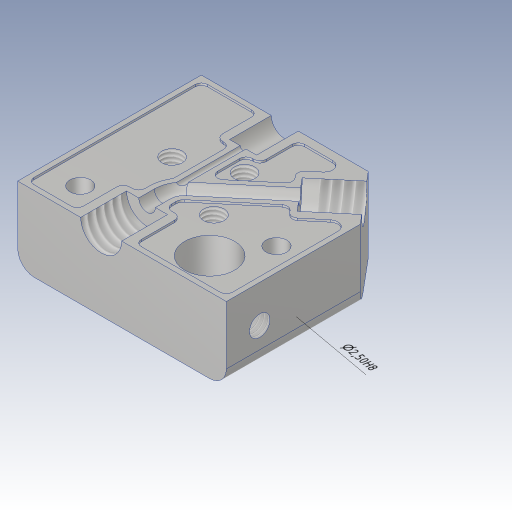
# Autodesk Inventor part: BT001_huenin20_23
Saved by Autodesk Inventor 2023.3 (Build 273359000, 359)
## iProperties
Company: HTBLA Kaindorf
RuleStatus: InUse
Created: 2023-05-23
Part Number: BT001_huenin20_23
Project: Fiberprinter-Hotend
Material: Aluminium
Description: Heizblock_Seite1
Document SubType Name: Modeling
Designer: huenin20
Density: 2.7 g/cm^3
Appearance: Aluminium - flach
Mass: 10.9063 g
Surface Area: 24.2904 cm^2
Volume: 4.03936 cm^3
AfterDocNew0: iProperties-Editor_aufrufen
Author: nicob
Keywords: 2023
Autodesk Inventor part; units mm, degrees
ref_plane "YZ Plane" through (0, 0, 0) normal (1, 0, 0) x (0, 1, 0)
ref_plane "XZ Plane" through (0, 0, 0) normal (0, 1, 0) x (-1, 0, 0)
ref_plane "XY Plane" through (0, 0, 0) normal (0, 0, 1) x (1, 0, 0)
sketch "Skizze3" plane through (0, 0, 0) normal (0, 0, 1) x (1, 0, 0)
  line L0 (0, 0) -> (-22, 0)
  line L1 (-16.0412, 25) -> (0, 25)
  line L2 (0, 25) -> (0, 0)
  circle A0 centre (-4, 19) radius 3
  line L3 (-22, 20) -> (-16.0412, 25)
  line L4 (-22, 20) -> (-22, 0)
  line L5 (-19.0206, 22.5) -> (-9.2812, 10.893)
  arc A1 (-9.2812, 10.893) -> (-7.3661, 10) centre (-7.3661, 12.5) ccw
  line L6 (-7.3661, 10) -> (0, 10)
  dimension "d115" = 6
  dimension "d116" = 6
  dimension "d117" = 4
  dimension "d234" = 130
  dimension "d236" = 25
  dimension "d237" = 22
  dimension "d238" = 2.5
  dimension "d306" = 15
  dimension "d325" = 20
  constraints: 15 end point, 2 centre point, 2 perpendicular, 2 point on circle, 2 tangent, 1 horizontal, 1 midpoint, 1 parallel, 1 point on line
  measures "d115" diameter of A0
  measures "d116" distance from line of L1 A0.centre
  measures "d117" distance from line of L2 A0.centre
  measures "d234" angle of L4 L3
  measures "d236" distance between parallel lines of L1 L0
  measures "d237" distance between parallel lines of L2 L4
  measures "d238" radius of A1
  measures "d306" distance between parallel lines of L1 L6
  measures "d325" distance of L3.start L0.end
extrude "Extrusion11" add sketch "Skizze3" against normal blind 9
sketch "Skizze19" plane through (-22, 20, -9) normal (-0.6427876, 0.7660444, 0) x (0.7660444, 0.6427876, 0)
  circle A0 centre (3.8893, -9) radius 1
  point P0 (3.9972, -9)
  dimension "d241" = 2
  constraints: 1 centre point, 1 coincident
  measures "d241" diameter of A0
sweep "Sweeping4" cut profiles "Skizze19" path "Skizze3" path curves L5 A1 L6
hole "Bohrung17" at (-19.0206, 22.5, 0) direction (0.6427876, -0.7660444, 0) diameter 4.917 depth 5.5
sketch "Skizze20" plane through (0, 0, -9) normal (1, 0, 0) x (0, 0, -1)
  arc A0 (-9, 9) -> (-9, 11) centre (-9, 10) ccw projected
  point P0 (-9, 0)
hole "Bohrung18" at (0, 10, 0) direction (-1, 0, 0) diameter 4.917 depth 5.5
hole "Bohrung27" at (0, 10, 0) direction (-1, 0, 0) diameter 0.7 depth 11
sketch "Skizze21" plane through (-22, 0, 0) normal (-1, 0, 0) x (0, 0, 1)
  arc A0 (0, 11) -> (0, 9) centre (0, 10) ccw projected
  line L0 (0, 20) -> (0, 0) projected
  line L1 (0, 10.35) -> (-0.35, 10)
  line L2 (-0.35, 10) -> (0, 9.65)
  line L3 (0, 9.65) -> (0, 10.35) projected
  arc A1 (0, 10.35) -> (0, 9.65) centre (0, 10) ccw projected
  point P0 (0, 10)
  point P1 (-0.35, 10)
  point P2 (-0.35, 10)
  point P3 (0, 9.65)
  dimension "d345" = 45
  dimension "d347" = 0.7
  constraints: 4 end point, 2 point on line, 1 horizontal alignment, 1 midpoint, 1 perpendicular
  measures "d345" angle of L0 L2
  measures "d347" distance of L1.start L2.end
hole "Bohrung20" at (-22, 10, 0) direction (1, 0, 0) diameter 3.242 depth 5
sketch "Skizze22" plane through (0, 0, 0) normal (0, 0, 1) x (1, 0, 0)
  line L0 (0, 7.5415) -> (-5.5, 7.5415) projected
  line L1 (0, 12.4585) -> (0, 7.5415) projected
  line L2 (-5.5, 12.4585) -> (0, 12.4585) projected
  line L3 (-5.5, 7.5415) -> (-5.5, 12.4585) projected
  line L4 (-5.5, 10) -> (-7.3661, 10)
  line L5 (-7.3661, 9) -> (-7.3661, 11) projected
  line L6 (-6, 10) -> (-6, 11.5)
  line L7 (-6, 11.5) -> (-7, 11.5)
  line L8 (-7, 11.5) -> (-7, 10)
  point P0 (0, 0)
  dimension "d273" = 1
  dimension "d274" = 0.5
  dimension "d275" = 3
  constraints: 8 end point, 2 midpoint, 2 perpendicular, 2 point on line, 1 vertical
  measures "d273" distance of L6.end L7.end
  measures "d274" distance between parallel lines of L3 L6
  measures "d275" diameter of L7 L4
revolve "Umdrehung2" [suppressed]
sketch "Skizze23" plane through (0, 25, -9) normal (0, 1, 0) x (0, 0, -1)
  line L0 (0, 7) -> (0, 1) projected
  line L1 (-9, 1) -> (-9, 7) projected
  line L2 (-9, 0) -> (0, 0) projected
  point P0 (-4.5, 4)
  point P1 (-9, 4)
  point P2 (-4.5, 0)
  constraints: 2 midpoint, 1 horizontal alignment, 1 vertical alignment
hole "Bohrung28" at (-4, 25, -4.5) direction (0, -1, 0) diameter 2.459 depth 6 tip angle 118
sketch "Skizze24" plane through (0, 0, 0) normal (0, 0, 1) x (1, 0, 0)
  line L0 (-7.3661, 11) -> (-5.5, 11) projected
  line L1 (-5.5, 11) -> (-5.5, 12.4585) projected
  line L2 (-5.5, 12.4585) -> (0, 12.4585) projected
  line L3 (0, 12.4585) -> (0, 25) projected
  line L4 (0, 25) -> (-16.0412, 25) projected
  circle A0 centre (-4, 19) radius 3 projected
  line L5 (-16.0412, 25) -> (-17.1373, 24.0803) projected
  line L6 (-17.1373, 24.0803) -> (-13.602, 19.867) projected
  line L7 (-13.602, 19.867) -> (-14.7192, 18.9295) projected
  line L8 (-14.7192, 18.9295) -> (-8.5152, 11.5358) projected
  arc A1 (-8.5152, 11.5358) -> (-7.3661, 11) centre (-7.3661, 12.5) ccw projected
  line L9 (-5.5, 9) -> (-7.3661, 9) projected
  arc A2 (-9.3977, 9.65) -> (-7.3661, 9) centre (-7.3661, 12.5) ccw projected
  line L10 (-10.131, 10.35) -> (-16.2513, 17.644) projected
  line L11 (-16.2513, 17.644) -> (-17.3686, 16.7065) projected
  line L12 (-17.3686, 16.7065) -> (-20.9039, 20.9197) projected
  line L13 (-20.9039, 20.9197) -> (-22, 20) projected
  line L14 (-22, 20) -> (-22, 11.621) projected
  line L15 (-22, 11.621) -> (-17, 11.621) projected
  line L16 (-17, 11.621) -> (-17, 8.379) projected
  line L17 (-17, 8.379) -> (-22, 8.379) projected
  line L18 (-22, 8.379) -> (-22, 0) projected
  line L19 (-22, 0) -> (0, 0) projected
  line L20 (0, 0) -> (0, 7.5415) projected
  line L21 (0, 7.5415) -> (-5.5, 7.5415) projected
  line L22 (-5.5, 7.5415) -> (-5.5, 9) projected
  line L23 (-9.3977, 9.65) -> (-11, 9.65) projected
  line L24 (-11, 9.65) -> (-11, 10.35) projected
  line L25 (-11, 10.35) -> (-10.131, 10.35) projected
  point P0 (-14.7, 12.48)
  point P1 (-9, 22)
  point P2 (-8.5, 15)
  point P3 (-12, 6.5)
  point P4 (-3.5, 4)
  dimension "d343" = 7.3
  dimension "d344" = 13
  dimension "d357" = 6.5
  dimension "d358" = 10
  dimension "d359" = 4
  dimension "d360" = 3.5
  dimension "d381" = 12.48
  dimension "d382" = 3
  dimension "d383" = 10
  dimension "d384" = 8.5
  measures "d343" distance from line of L14 point (-14.7, 12.48)
  measures "d344" distance from line of L14 point (-9, 22)
  measures "d357" distance from line of L19 point (-12, 6.5)
  measures "d358" distance from line of L18 point (-12, 6.5)
  measures "d359" distance from line of L19 point (-3.5, 4)
  measures "d360" distance from line of L20 point (-3.5, 4)
  measures "d381" distance from line of L19 point (-14.7, 12.48)
  measures "d382" distance from line of L4 point (-9, 22)
  measures "d383" distance from line of L4 point (-8.5, 15)
  measures "d384" distance from line of L3 point (-8.5, 15)
hole "Bohrung23" at (-9, 22, 0) at (-3.5, 4, 0) direction (0, 0, -1) diameter 2.5 end through all
fillet "Rundung5" radius 2 2 edges at (-11, 0, -9) (-8.0206, 25, -9)
hole "Bohrung24" at (-8.5, 15, 0) at (-12, 6.5, 0) at (-14.7, 12.48, 0) direction (0, 0, -1) diameter 2.459 end through all
sketch "Skizze25" plane through (-22, 20, -9) normal (-1, 0, 0) x (0, 0, 1)
  arc A0 (0, -18) -> (2, -20) centre (2, -18) ccw projected
  line L0 (9, -20) -> (2, -20) projected
  line L1 (9, -11.621) -> (9, -20) projected
  arc A1 (9, -8.379) -> (9, -11.621) centre (9, -10) ccw projected
  line L2 (9, 0) -> (9, -8.379) projected
  line L3 (9, 0) -> (0, 0) projected
  line L4 (0, -18) -> (0, 0) projected
  line L5 (2.5, -16) -> (2.5, -4) construction
  point P0 (9, -20)
  point P1 (2.5, -10)
  point P2 (2.5, -10)
  dimension "d326" = 4
  dimension "d327" = 4
  dimension "d328" = 2.5
  dimension "d361" = 0
  constraints: 2 coincident, 2 end point, 1 midpoint, 1 vertical, 1 vertical alignment
  measures "d326" distance from line of L0 L5.start
  measures "d327" distance from line of L3 point (2.5, -4)
  measures "d328" distance from line of L4 point (2.5, -4)
  measures "d361" distance from line of L5 point (2.5, -10)
hole "Bohrung25" at (-22, 4, -6.5) at (-22, 16, -6.5) direction (1, 0, 0) diameter 2.5 depth 3.5
hole "Bohrung26" at (-22, 10, -6.5) direction (1, 0, 0) diameter 1.567 depth 4 tip angle 118
extrude "Extrusion12" cut sketch "Skizze21" against normal blind 15 contours L0 L2 L1 | L1 A1 | A1 L2
sketch "Skizze27" plane through (0, 0, 0) normal (0, 0, 1) x (1, 0, 0)
  line L0 (-5.5, 11) -> (-5.5, 12.4585) projected
  line L1 (-5.5, 12.4585) -> (0, 12.4585) projected
  line L2 (0, 12.4585) -> (0, 25) projected
  line L3 (0, 25) -> (-16.0412, 25) projected
  line L4 (-16.0412, 25) -> (-17.1373, 24.0803) projected
  line L5 (-17.1373, 24.0803) -> (-13.602, 19.867) projected
  line L6 (-13.602, 19.867) -> (-14.7192, 18.9295) projected
  line L7 (-14.7192, 18.9295) -> (-8.5152, 11.5358) projected
  arc A0 (-8.5152, 11.5358) -> (-7.3661, 11) centre (-7.3661, 12.5) ccw projected
  line L8 (-7.3661, 11) -> (-5.5, 11) projected
  line L9 (-9.3977, 9.65) -> (-17, 9.65) projected
  line L10 (-17, 9.65) -> (-17, 8.379) projected
  line L11 (-17, 8.379) -> (-22, 8.379) projected
  line L12 (-22, 8.379) -> (-22, 0) projected
  line L13 (-22, 0) -> (0, 0) projected
  line L14 (0, 0) -> (0, 7.5415) projected
  line L15 (0, 7.5415) -> (-5.5, 7.5415) projected
  line L16 (-5.5, 7.5415) -> (-5.5, 9) projected
  line L17 (-5.5, 9) -> (-7.3661, 9) projected
  arc A1 (-9.3977, 9.65) -> (-7.3661, 9) centre (-7.3661, 12.5) ccw projected
  line L18 (-17, 10.35) -> (-10.131, 10.35) projected
  line L19 (-10.131, 10.35) -> (-16.2513, 17.644) projected
  line L20 (-16.2513, 17.644) -> (-17.3686, 16.7065) projected
  line L21 (-17.3686, 16.7065) -> (-20.9039, 20.9197) projected
  line L22 (-20.9039, 20.9197) -> (-22, 20) projected
  line L23 (-22, 20) -> (-22, 11.621) projected
  line L24 (-22, 11.621) -> (-17, 11.621) projected
  line L25 (-17, 11.621) -> (-17, 10.35) projected
  circle A2 centre (-14.7, 12.48) radius 1.2295 projected
  line L26 (-20.65, 7.379) -> (-17.15, 7.379)
  line L27 (-16.4, 8.129) -> (-16.4, 8.3)
  line L28 (-15.65, 9.05) -> (-9.7915, 9.05)
  arc A3 (-9.4164, 8.9495) -> (-7.3661, 8.4) centre (-7.3661, 12.5) ccw
  line L29 (-7.3661, 8.4) -> (-6.85, 8.4)
  line L30 (-6.1, 7.65) -> (-6.1, 7.2915)
  line L31 (-5.35, 6.5415) -> (-1.35, 6.5415)
  line L32 (-0.6, 5.7915) -> (-0.6, 1.35)
  line L33 (-1.35, 0.6) -> (-20.65, 0.6)
  line L34 (-21.4, 1.35) -> (-21.4, 6.629)
  line L35 (-21, 13.371) -> (-21, 19.5337)
  line L36 (-21, 19.5337) -> (-21.0272, 19.5109)
  line L37 (-21.0272, 19.5109) -> (-18.2311, 16.1786)
  line L38 (-17.1744, 16.0861) -> (-16.8998, 16.3166)
  line L39 (-15.8432, 16.2241) -> (-12.4515, 12.1821)
  line L40 (-13.026, 10.95) -> (-15.65, 10.95)
  line L41 (-16.4, 11.7) -> (-16.4, 11.871)
  line L42 (-17.15, 12.621) -> (-20.25, 12.621)
  line L43 (-8.0555, 11.9215) -> (-13.3918, 18.2811)
  line L44 (-13.2994, 19.3377) -> (-13.0248, 19.5681)
  line L45 (-12.9323, 20.6247) -> (-15.9856, 24.2635)
  line L46 (-15.9856, 24.2635) -> (-15.8228, 24.4)
  line L47 (-15.8228, 24.4) -> (-1.35, 24.4)
  line L48 (-0.6, 23.65) -> (-0.6, 14.2085)
  line L49 (-1.35, 13.4585) -> (-5.35, 13.4585)
  line L50 (-6.1, 12.7085) -> (-6.1, 12.35)
  line L51 (-6.85, 11.6) -> (-7.3661, 11.6)
  arc A4 (-8.0555, 11.9215) -> (-7.3661, 11.6) centre (-7.3661, 12.5) ccw
  arc A5 (-19.234, 17.3738) -> (-21, 16.731) centre (-20, 16.731) ccw
  arc A6 (-13.9556, 24.4) -> (-14.7217, 22.7572) centre (-13.9556, 23.4) ccw
  arc A7 (-16.4, 11.7) -> (-15.65, 10.95) centre (-15.65, 11.7) ccw
  arc A8 (-13.026, 10.95) -> (-12.4515, 12.1821) centre (-13.026, 11.7) ccw
  arc A9 (-15.8432, 16.2241) -> (-16.8998, 16.3166) centre (-16.4177, 15.742) ccw
  arc A10 (-21, 13.371) -> (-20.25, 12.621) centre (-20.25, 13.371) ccw
  arc A11 (-13.2994, 19.3377) -> (-13.3918, 18.2811) centre (-12.8173, 18.7631) ccw
  arc A12 (-6.85, 11.6) -> (-6.1, 12.35) centre (-6.85, 12.35) ccw
  arc A13 (-1.35, 13.4585) -> (-0.6, 14.2085) centre (-1.35, 14.2085) ccw
  arc A14 (-0.6, 23.65) -> (-1.35, 24.4) centre (-1.35, 23.65) ccw
  arc A15 (-6.1, 7.65) -> (-6.85, 8.4) centre (-6.85, 7.65) ccw
  arc A16 (-9.4164, 8.9495) -> (-9.7915, 9.05) centre (-9.7915, 8.3) ccw
  arc A17 (-15.65, 9.05) -> (-16.4, 8.3) centre (-15.65, 8.3) ccw
  arc A18 (-20.65, 7.379) -> (-21.4, 6.629) centre (-20.65, 6.629) ccw
  arc A19 (-21.4, 1.35) -> (-20.65, 0.6) centre (-20.65, 1.35) ccw
  arc A20 (-1.35, 0.6) -> (-0.6, 1.35) centre (-1.35, 1.35) ccw
  arc A21 (-0.6, 5.7915) -> (-1.35, 6.5415) centre (-1.35, 5.7915) ccw
  arc A22 (-6.1, 7.2915) -> (-5.35, 6.5415) centre (-5.35, 7.2915) ccw
  arc A23 (-17.15, 7.379) -> (-16.4, 8.129) centre (-17.15, 8.129) ccw
  arc A24 (-16.4, 11.871) -> (-17.15, 12.621) centre (-17.15, 11.871) ccw
  arc A25 (-18.2311, 16.1786) -> (-17.1744, 16.0861) centre (-17.6565, 16.6607) ccw
  arc A26 (-13.0248, 19.5681) -> (-12.9323, 20.6247) centre (-13.5069, 20.1427) ccw
  arc A27 (-5.35, 13.4585) -> (-6.1, 12.7085) centre (-5.35, 12.7085) ccw
  point P0 (-9.5814, 9.05)
  dimension "d400" = 0.6
  dimension "d401" = 0.6
  dimension "d402" = 1
  dimension "d403" = 1
  dimension "d404" = 1
  dimension "d405" = 0.6
  dimension "d406" = 0.6
  dimension "d407" = 0.6
  dimension "d408" = 0.6
  dimension "d409" = 1
  dimension "d410" = 1
  dimension "d411" = 1
  dimension "d412" = 1
  dimension "d413" = 1
  dimension "d414" = 0.75
  constraints: 52 end point, 51 point on circle, 46 tangent, 27 centre point, 20 equal radius, 5 point on line, 16 other
  measures "d400" distance between parallel lines of L13 L33
  measures "d401" distance between parallel lines of L18 L40
  measures "d402" distance between parallel lines of L24 L42
  measures "d403" distance between parallel lines of L21 L37
  measures "d404" distance between parallel lines of L11 L26
  measures "d405" distance between parallel lines of L9 L28
  measures "d406" distance between parallel lines of L3 L47
  measures "d407" distance between parallel lines of L7 L43
  measures "d408" distance between parallel lines of L8 L51
  measures "d409" distance between parallel lines of L5 L45
  measures "d410" distance between parallel lines of L1 L49
  measures "d411" distance between parallel lines of L15 L31
  measures "d412" radius of A6
  measures "d413" radius of A5
  measures "d414" radius of A7
extrude "Extrusion14" cut sketch "Skizze27" against normal blind 0.25 contours L26 A23 L27 A17 L28 A16 A3 L29 A15 L30 A22 L31 A21 L32 A20 L33 A19 L34 A18 | L35 A5 L37 A25 L38 A9 L39 A8 L40 A7 L41 A24 L42 A10 | L43 A11 L44 A26 L45 A6 L47 A14 L48 A13 L49 A27 L50 A12 L51 A4
equation "\"Heizpatronen_durchmesser\" = 6"
